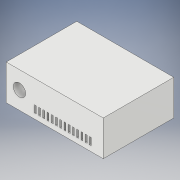
# Autodesk Inventor part: Head
Saved by Autodesk Inventor 2017 SP1 (Build 210196100, 196)
## iProperties
Created: 2018-02-11
Part Number: Head
Material: ABS Plastic
Document SubType Name: Modeling
Designer: Zach
Density: 1.06 g/cm^3
Appearance: CR White
Author: Zach
Autodesk Inventor part; units mm, degrees
ref_plane "YZ Plane" through (0, 0, 0) normal (1, 0, 0) x (0, 1, 0)
ref_plane "XZ Plane" through (0, 0, 0) normal (0, 1, 0) x (-1, 0, 0)
ref_plane "XY Plane" through (0, 0, 0) normal (0, 0, 1) x (1, 0, 0)
sketch "Sketch1" plane through (0, 0, 0) normal (0, 0, 1) x (1, 0, 0)
  line L0 (0, 0) -> (27.5, 0)
  line L1 (27.5, 0) -> (27.5, 10)
  line L2 (27.5, 10) -> (0, 10)
  line L3 (0, 10) -> (0, 0)
  dimension "d0" = 27.5
  dimension "d1" = 10
  constraints: 8 end point, 2 parallel, 1 horizontal, 1 perpendicular
  measures "d0" distance of L2.end L1.end
  measures "d1" distance of L1.end L0.end
extrude "Extrusion1" add sketch "Sketch1" along normal blind 20
sketch "Sketch2" plane through (0, 0, 20) normal (0, 0, 1) x (1, 0, 0)
  circle A0 centre (3.75, 5) radius 1.75
  line L0 (0, 0) -> (27.5, 0) projected
  line L1 (0, 10) -> (0, 0) projected
  line L2 (24.1, 3.5) -> (23.6, 3.5)
  line L3 (23.6, 3.5) -> (23.6, 1.5)
  line L4 (23.6, 1.5) -> (24.1, 1.5)
  line L5 (24.1, 1.5) -> (24.1, 3.5)
  line L6 (27.5, 0) -> (27.5, 10) projected
  line L7 (22.9, 3.5) -> (22.4, 3.5)
  line L8 (22.4, 3.5) -> (22.4, 1.5)
  line L9 (22.4, 1.5) -> (22.9, 1.5)
  line L10 (22.9, 1.5) -> (22.9, 3.5)
  line L11 (21.7, 3.5) -> (21.2, 3.5)
  line L12 (21.2, 3.5) -> (21.2, 1.5)
  line L13 (21.2, 1.5) -> (21.7, 1.5)
  line L14 (21.7, 1.5) -> (21.7, 3.5)
  line L15 (20.5, 3.5) -> (20, 3.5)
  line L16 (20, 3.5) -> (20, 1.5)
  line L17 (20, 1.5) -> (20.5, 1.5)
  line L18 (20.5, 1.5) -> (20.5, 3.5)
  line L19 (19.3, 3.5) -> (18.8, 3.5)
  line L20 (18.8, 3.5) -> (18.8, 1.5)
  line L21 (18.8, 1.5) -> (19.3, 1.5)
  line L22 (19.3, 1.5) -> (19.3, 3.5)
  line L23 (18.1, 3.5) -> (17.6, 3.5)
  line L24 (17.6, 3.5) -> (17.6, 1.5)
  line L25 (17.6, 1.5) -> (18.1, 1.5)
  line L26 (18.1, 1.5) -> (18.1, 3.5)
  line L27 (16.9, 3.5) -> (16.4, 3.5)
  line L28 (16.4, 3.5) -> (16.4, 1.5)
  line L29 (16.4, 1.5) -> (16.9, 1.5)
  line L30 (16.9, 1.5) -> (16.9, 3.5)
  line L31 (15.7, 3.5) -> (15.2, 3.5)
  line L32 (15.2, 3.5) -> (15.2, 1.5)
  line L33 (15.2, 1.5) -> (15.7, 1.5)
  line L34 (15.7, 1.5) -> (15.7, 3.5)
  line L35 (14.5, 3.5) -> (14, 3.5)
  line L36 (14, 3.5) -> (14, 1.5)
  line L37 (14, 1.5) -> (14.5, 1.5)
  line L38 (14.5, 1.5) -> (14.5, 3.5)
  line L39 (13.3, 3.5) -> (12.8, 3.5)
  line L40 (12.8, 3.5) -> (12.8, 1.5)
  line L41 (12.8, 1.5) -> (13.3, 1.5)
  line L42 (13.3, 1.5) -> (13.3, 3.5)
  line L43 (12.1, 3.5) -> (11.6, 3.5)
  line L44 (11.6, 3.5) -> (11.6, 1.5)
  line L45 (11.6, 1.5) -> (12.1, 1.5)
  line L46 (12.1, 1.5) -> (12.1, 3.5)
  line L47 (10.9, 3.5) -> (10.4, 3.5)
  line L48 (10.4, 3.5) -> (10.4, 1.5)
  line L49 (10.4, 1.5) -> (10.9, 1.5)
  line L50 (10.9, 1.5) -> (10.9, 3.5)
  line L51 (9.7, 3.5) -> (9.2, 3.5)
  line L52 (9.2, 3.5) -> (9.2, 1.5)
  line L53 (9.2, 1.5) -> (9.7, 1.5)
  line L54 (9.7, 1.5) -> (9.7, 3.5)
  line L55 (8.5, 3.5) -> (8, 3.5)
  line L56 (8, 3.5) -> (8, 1.5)
  line L57 (8, 1.5) -> (8.5, 1.5)
  line L58 (8.5, 1.5) -> (8.5, 3.5)
  dimension "d4" = 5
  dimension "d5" = 3.75
  dimension "d6" = 3.5
  dimension "d7" = 0.5
  dimension "d8" = 2
  dimension "d9" = 3.4
  dimension "d10" = 1.5
  dimension "d13" = 1.2
  constraints: 112 end point, 2 horizontal, 2 parallel, 1 centre point, 1 perpendicular, 104 other
  measures "d4" distance from line of L0 A0.centre
  measures "d5" distance from line of L1 A0.centre
  measures "d6" diameter of A0
  measures "d7" distance of L2.start L2.end
  measures "d8" distance of L4.end L2.start
  measures "d9" distance between parallel lines of L6 L5
  measures "d10" distance between parallel lines of L0 L4
  measures "d13" distance of L2.start L7.start
extrude "Extrusion2" cut sketch "Sketch2" against normal blind 3
body "Solid1"
